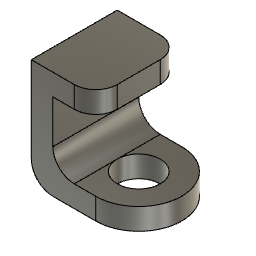
exercise 3 v2 (Autodesk Fusion 360 design; units mm, degrees)
Autodesk Fusion 360 part; units mm, degrees
note: some values were not read from the file. Set by a fixed rule: which sketch regions a step uses.
sketch "Sketch1" plane through (0, 0, 0) normal (0, 0, 1) x (1, 0, 0)
  line L0 (0, 0) -> (30, 0)
  line L1 (30, 0) -> (30, -40)
  line L2 (30, -40) -> (0, -40)
  line L3 (0, -40) -> (0, 0)
  circle A0 centre (30, -20) radius 20
  circle A1 centre (30, -20) radius 10
  dimension "d1" = 30
  dimension "d2" = 40
  dimension "d3" = 40
  dimension "d4" = 20
  constraint horizontal L0
  constraint vertical L1
  constraint horizontal L2
  constraint vertical L3
  constraint coincident L0.start L3.end
  constraint midpoint L1 A0.centre
  constraint concentric A0 A1
  measures "d1" distance of L0.start L0.end
  measures "d2" distance of L0.start L2.end
  measures "d3" diameter of A0
  measures "d4" diameter of A1
extrude "Extrude1" add sketch "Sketch1" along normal blind 10 contours L0 L2 L3 A0 | L1 A0 A1 | L1 A0 A1
sketch "Sketch2" plane through (0, 0, 0) normal (0, 1, 0) x (1, 0, 0)
sketch "Sketch3" plane through (0, -40, 0) normal (0, -1, 0) x (1, 0, 0)
  line L0 (0, 0) -> (30, 0)
  line L1 (30, 0) -> (30, 10)
  line L2 (30, 10) -> (0, 10)
  line L3 (0, 10) -> (0, 0)
  line L4 (0, 0) -> (0, 50.06)
  line L5 (0, 50.06) -> (30, 50.06)
  line L6 (30, 50.06) -> (30, 40.06)
  line L7 (30, 40.06) -> (10, 40.06)
  line L8 (10, 40.06) -> (10, 0)
  dimension "d7" = 10
  dimension "d8" = 30
  dimension "d10" = 10
  dimension "d11" = 50.06
  constraint coincident L0.start L3.end
  constraint perpendicular L0 L4
  constraint perpendicular L3 L5
  constraint perpendicular L5 L6
  constraint perpendicular L3 L7
  constraint coincident L0 L8.end
  constraint perpendicular L0 L8
  measures "d7" distance of L4 L8
  measures "d8" distance of L4 L6
  measures "d10" distance of L5 L7
  measures "d11" distance of L0 L5
extrude "Extrude2" add sketch "Sketch3" against normal blind 40 contours L2 L4 L5 L6 L7 L8
fillet "Fillet1" radius 10 1 edges at (30, -40, 45.06)
fillet "Fillet2" radius 10 1 edges at (30, 0, 45.06)
fillet "Fillet3" radius 10 1 edges at (0, -20, 0)
fillet "Fillet4" radius 10 1 edges at (10, -20, 10)
